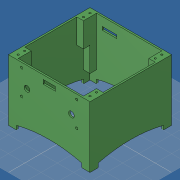
# Autodesk Inventor part: DayLightGlow_Base
Saved by Autodesk Inventor 2019 (Build 230136000, 136)
## iProperties
Created: 2019-01-03
Part Number: DayLightGlow_Base
Material: Generisch
Document SubType Name: Modeling
Designer: Stefan
Mass: 74.5132 g
Surface Area: 583.544 cm^2
Volume: 74.5132 cm^3
Density: 1 g/cm^3
Appearance: Glatt - waldgrün
Author: Stefan
Autodesk Inventor part; units mm, degrees
ref_plane "YZ Plane" through (0, 0, 0) normal (1, 0, 0) x (0, 1, 0)
ref_plane "XZ Plane" through (0, 0, 0) normal (0, 1, 0) x (-1, 0, 0)
ref_plane "XY Plane" through (0, 0, 0) normal (0, 0, 1) x (1, 0, 0)
sketch "Skizze1" plane through (0, 0, 0) normal (0, 1, 0) x (-1, 0, 0)
  line L0 (-50, 50) -> (50, 50)
  line L1 (50, 50) -> (50, -50)
  line L2 (50, -50) -> (-50, -50)
  line L3 (-50, -50) -> (-50, 50)
  line L4 (-50, 50) -> (50, -50) construction
  line L5 (50, 50) -> (-50, -50) construction
  point P0 (0, 0)
  dimension "d0" = 100
  dimension "d1" = 100
  constraints: 12 end point, 2 midpoint, 2 parallel, 1 horizontal, 1 perpendicular
  measures "d0" distance of L0.end L1.end
  measures "d1" distance of L0.start L0.end
extrude "Extrusion1" add sketch "Skizze1" along normal blind 75
sketch "Skizze2" plane through (0, 0, 0) normal (1, 0, 0) x (0, 1, 0)
  line L0 (5, 40) -> (0, 40)
  line L1 (0, 40) -> (0, -40)
  line L2 (0, -40) -> (5, -40)
  arc A0 (5, -40) -> (5, 40) centre (-152.5, 0) ccw
  point P0 (0, 0)
  point P1 (0, 0)
  dimension "d4" = 5
  dimension "d6" = 80
  dimension "d30" = 10
  constraints: 6 end point, 2 perpendicular, 2 point on circle, 1 centre point, 1 coincident, 1 horizontal, 1 midpoint, 1 parallel
  measures "d4" distance of L0.start L0.end
  measures "d6" distance between parallel lines of L2 L0
  measures "d30" distance edge to line of A0 L1
extrude "Extrusion2" cut sketch "Skizze2" along normal through all both and the other way through all
sketch "Skizze3" plane through (0, 0, 0) normal (0, 0, 1) x (1, 0, 0)
  line L0 (-40, 5) -> (-40, 0)
  line L1 (-40, 0) -> (40, 0)
  line L2 (40, 0) -> (40, 5)
  arc A0 (40, 5) -> (-40, 5) centre (0, -152.5) ccw
  point P0 (0, 0)
  point P1 (0, 0)
  point P2 (0, 0)
  dimension "d9" = 5
  dimension "d11" = 80
  dimension "d29" = 10
  constraints: 6 end point, 2 coincident, 2 perpendicular, 2 point on circle, 1 centre point, 1 horizontal, 1 midpoint, 1 parallel
  measures "d9" distance of L0.start L0.end
  measures "d11" distance between parallel lines of L2 L0
  measures "d29" distance edge to line of A0 L1
extrude "Extrusion3" cut sketch "Skizze3" along normal through all both and the other way through all
sketch "Skizze9" plane through (0, 75, 0) normal (0, 1, 0) x (1, 0, 0)
  line L0 (-50, -50) -> (50, -50) projected
  line L1 (50, -50) -> (50, 50) projected
  line L2 (50, 50) -> (-50, 50) projected
  line L3 (-50, 50) -> (-50, -50) projected
  line L4 (-48, -48) -> (48, -48)
  line L5 (48, -48) -> (48, 48)
  line L6 (48, 48) -> (-48, 48)
  line L7 (-48, 48) -> (-48, -48)
  line L8 (-40, 40) -> (-48, 40)
  line L9 (-48, 40) -> (-48, 48)
  line L10 (-48, 48) -> (-40, 48)
  line L11 (-40, 48) -> (-40, 40)
  line L12 (-40, 40) -> (-48, 48) construction
  line L13 (-48, 40) -> (-40, 48) construction
  line L14 (40, 40) -> (48, 40)
  line L15 (48, 40) -> (48, 48)
  line L16 (48, 48) -> (40, 48)
  line L17 (40, 48) -> (40, 40)
  line L18 (40, 40) -> (48, 48) construction
  line L19 (48, 40) -> (40, 48) construction
  line L20 (40, -40) -> (48, -40)
  line L21 (48, -40) -> (48, -48)
  line L22 (48, -48) -> (40, -48)
  line L23 (40, -48) -> (40, -40)
  line L24 (40, -40) -> (48, -48) construction
  line L25 (48, -40) -> (40, -48) construction
  line L26 (40, -32) -> (48, -32)
  line L27 (48, -32) -> (48, -40)
  line L28 (48, -40) -> (40, -40)
  line L29 (40, -40) -> (40, -32)
  line L30 (40, -32) -> (48, -40) construction
  line L31 (48, -32) -> (40, -40) construction
  line L32 (-40, 32) -> (-48, 32)
  line L33 (-48, 32) -> (-48, 40)
  line L34 (-48, 40) -> (-40, 40)
  line L35 (-40, 40) -> (-40, 32)
  line L36 (-40, 32) -> (-48, 40) construction
  line L37 (-48, 32) -> (-40, 40) construction
  line L38 (40, 32) -> (48, 32)
  line L39 (48, 32) -> (48, 40)
  line L40 (48, 40) -> (40, 40)
  line L41 (40, 40) -> (40, 32)
  line L42 (40, 32) -> (48, 40) construction
  line L43 (48, 32) -> (40, 40) construction
  line L44 (-40, -40) -> (-48, -40)
  line L45 (-48, -40) -> (-48, -48)
  line L46 (-48, -48) -> (-40, -48)
  line L47 (-40, -48) -> (-40, -40)
  line L48 (-40, -40) -> (-48, -48) construction
  line L49 (-48, -40) -> (-40, -48) construction
  line L50 (-40, -32) -> (-48, -32)
  line L51 (-48, -32) -> (-48, -40)
  line L52 (-48, -40) -> (-40, -40)
  line L53 (-40, -40) -> (-40, -32)
  line L54 (-40, -32) -> (-48, -40) construction
  line L55 (-48, -32) -> (-40, -40) construction
  point P0 (0, 0)
  point P1 (-44, 44)
  point P2 (44, 44)
  point P3 (44, -44)
  point P4 (44, -36)
  point P5 (-44, 36)
  point P6 (44, 36)
  point P7 (-44, -44)
  point P8 (-44, -36)
  point P9 (-44, 44)
  point P10 (-44, 36)
  point P11 (44, 44)
  point P12 (44, 36)
  point P13 (-44, -36)
  point P14 (-44, -44)
  point P15 (44, -36)
  point P16 (44, -44)
  dimension "d65" = 2
  dimension "d81" = 8
  dimension "d82" = 8
  constraints: 104 end point, 16 midpoint, 16 parallel, 14 collinear, 8 coincident, 8 horizontal, 8 perpendicular, 3 other
  measures "d65" distance between parallel lines of L3 L7
  measures "d81" distance between parallel lines of L10 L8
  measures "d82" distance between parallel lines of L11 L9
extrude "Extrusion9" cut sketch "Skizze9" against normal through all contours L7 L44 L47 L4 | L47 L53 L50 L7 L32 L35 L11 L6 L17 L41 L38 L5 L26 L29 L23 L4 | L7 L50 L53 L44 | L23 L20 L5 L4 | L29 L26 L5 L20 | L7 L8 L35 L32 | L7 L6 L11 L8 | L38 L41 L14 L5 | L14 L17 L6 L5
extrude "Extrusion10" add sketch "Skizze9" against normal blind 60 contours L7 L44 L47 L4 | L23 L20 L5 L4 | L7 L6 L11 L8 | L14 L17 L6 L5
extrude "Extrusion11" add sketch "Skizze9" against normal blind 30 contours L7 L50 L53 L44 | L29 L26 L5 L20 | L7 L8 L35 L32 | L38 L41 L14 L5
hole "Bohrung3" at (-44, 75, 44) at (-44, 75, 36) at (-44, 75, -36) at (-44, 75, -44) at (44, 75, -44) at (44, 75, -36) at (44, 75, 36) at (44, 75, 44) direction (0, -1, 0) diameter 2.2 end through all
sketch "Skizze10" plane through (0, -152.5, -48) normal (0, 0, 1) x (1, 0, 0)
  line L0 (-40, 227.5) -> (40, 227.5) projected
  circle A0 centre (30, 212) radius 3.25
  circle A1 centre (30, 200) radius 2.75
  line L1 (-33, 217) -> (-15, 217)
  line L2 (-15, 217) -> (-15, 213)
  line L3 (-15, 213) -> (-33, 213)
  line L4 (-33, 213) -> (-33, 217)
  line L5 (-33, 217) -> (-15, 213) construction
  line L6 (-15, 217) -> (-33, 213) construction
  line L7 (-48, 227.5) -> (-40, 227.5) projected
  line L8 (-48, 197.5) -> (-48, 227.5) projected
  line L9 (-40, 197.5) -> (-48, 197.5) projected
  line L10 (-40, 227.5) -> (-40, 197.5) projected
  line L11 (40, 227.5) -> (48, 227.5) projected
  line L12 (40, 227.5) -> (40, 197.5) projected
  line L13 (48, 197.5) -> (40, 197.5) projected
  line L14 (48, 227.5) -> (48, 197.5) projected
  point P0 (0, 152.5)
  point P1 (-24, 215)
  dimension "d83" = 6.5
  dimension "d84" = 15.5
  dimension "d85" = 18
  dimension "d86" = 5.5
  dimension "d87" = 2.5
  dimension "d89" = 15
  dimension "d90" = 18
  dimension "d91" = 4
  dimension "d92" = 15.5
  constraints: 12 end point, 2 centre point, 2 midpoint, 2 parallel, 1 horizontal, 1 perpendicular, 1 vertical alignment
  measures "d83" diameter of A0
  measures "d84" distance from line of L0 A0.centre
  measures "d85" distance from line of L14 A0.centre
  measures "d86" diameter of A1
  measures "d87" distance from line of L13 A1.centre
  measures "d89" distance between parallel lines of L4 L8
  measures "d90" distance of L1.start L1.end
  measures "d91" distance between parallel lines of L3 L1
  measures "d92" distance between parallel lines of L3 L9
extrude "Extrusion12" cut sketch "Skizze10" against normal up to surface (2 mm away) contours A0 | A1 | L1 L2 L3 L4
sketch "Skizze8" plane through (0, -142.5, 48) normal (0, 0, -1) x (-1, 0, 0)
  line L0 (-40, 217.5) -> (40, 217.5) projected
  line L1 (-7.5, 212.5) -> (7.5, 212.5)
  line L2 (7.5, 212.5) -> (7.5, 207.5)
  line L3 (7.5, 207.5) -> (-7.5, 207.5)
  line L4 (-7.5, 207.5) -> (-7.5, 212.5)
  circle A0 centre (27.3, 192.7) radius 3.4544 projected
  circle A1 centre (-27.3, 192.7) radius 3.5
  circle A2 centre (27.3, 192.7) radius 3.5
  circle A3 centre (-27.3, 192.7) radius 3.4544 projected
  circle A4 centre (-33.8, 211.8) radius 1.1 projected
  circle A5 centre (-33.8, 181.2) radius 1.1 projected
  circle A6 centre (33.8, 211.8) radius 1.1 projected
  circle A7 centre (33.8, 181.2) radius 1.1 projected
  circle A8 centre (-33.8, 211.8) radius 1.5
  circle A9 centre (33.8, 211.8) radius 1.5
  circle A10 centre (33.8, 181.2) radius 1.5
  circle A11 centre (-33.8, 181.2) radius 1.5
  point P0 (0, 152.5)
  point P1 (0, 212.5)
  point P2 (0, 217.5)
  point P3 (-40, 147.5)
  point P4 (40, 147.5)
  dimension "d57" = 15
  dimension "d58" = 5
  dimension "d59" = 5
  dimension "d60" = 7
  dimension "d61" = 7
  dimension "d64" = 3
  constraints: 8 end point, 6 centre point, 6 coincident, 3 equal radius, 2 midpoint, 2 parallel, 1 horizontal, 1 perpendicular, 1 vertical alignment
  measures "d57" distance between parallel lines of L2 L4
  measures "d58" distance between parallel lines of L3 L1
  measures "d59" distance between parallel lines of L1 L0
  measures "d60" diameter of A1
  measures "d61" diameter of A2
  measures "d64" diameter of A8
extrude "Extrusion8" cut sketch "Skizze8" against normal up to surface (2 mm away) contours L1 L2 L3 L4 | A0 | A1 | A2 | A3 | A4 | A5 | A6 | A7 | A8 | A9 | A10 | A11
